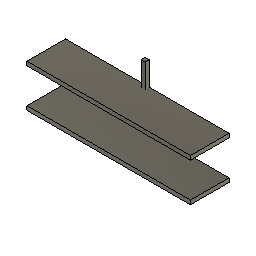
model (Autodesk Fusion 360 design; units mm, degrees)
Autodesk Fusion 360 part; units mm, degrees
sketch "front" plane through (0, 0, 0) normal (0, 1, 0) x (1, 0, 0) in component "shelf"
  line L0 (-10.5, -323.6094) -> (10.5, -323.6094)
  line L1 (10.5, -323.6094) -> (10.5, 200)
  line L2 (10.5, 200) -> (-10.5, 200)
  line L3 (-10.5, 200) -> (-10.5, -323.6094)
  line L4 (-423.6, -200) -> (423.6, -200)
  line L5 (423.6, -200) -> (423.6, -179)
  line L6 (423.6, -179) -> (-423.6, -179)
  line L7 (-423.6, -179) -> (-423.6, -200)
  line L8 (-423.6, 0) -> (423.6, 0)
  line L9 (423.6, 0) -> (423.6, 21)
  line L10 (423.6, 21) -> (-423.6, 21)
  line L11 (-423.6, 21) -> (-423.6, 0)
  line L12 (0, -200) -> (0, 0) construction
  line L13 (0, 0) -> (0, 200) construction
  line L14 (0, -200) -> (0, -323.6094) construction
  arc A0 (-180.0959, 31.5) -> (-217.05, 21) centre (-171.2117, -70.0461) ccw
  arc A1 (-99.149, 38.5819) -> (-10.5, 110.5) centre (-108.0332, 140.128) ccw
  line L15 (-180.0959, 31.5) -> (-99.149, 38.5819)
  line L16 (-10.5, 110.5) -> (10.5, 21) construction
  line L17 (-10.5, 110.5) -> (10.5, 200) construction
  line L18 (-423.6, 0) -> (-217.05, 21) construction
  line L19 (-10.5, 0) -> (-217.05, 21) construction
  arc A2 (-180.0959, -168.5) -> (-217.05, -179) centre (-171.2117, -270.0461) ccw
  line L20 (-180.0959, -168.5) -> (-99.149, -161.4181)
  arc A3 (-99.149, -161.4181) -> (-10.5, -89.5) centre (-108.0332, -59.872) ccw
  arc A4 (217.05, -179) -> (180.0959, -168.5) centre (171.2117, -270.0461) ccw
  line L21 (180.0959, -168.5) -> (99.149, -161.4181)
  arc A5 (10.5, -89.5) -> (99.149, -161.4181) centre (108.0332, -59.872) ccw
  arc A6 (217.05, 21) -> (180.0959, 31.5) centre (171.2117, -70.0461) ccw
  arc A7 (10.5, 110.5) -> (99.149, 38.5819) centre (108.0332, 140.128) ccw
  line L22 (180.0959, 31.5) -> (99.149, 38.5819)
  dimension "d1" = 200
  dimension "d2" = 123.6094
  dimension "d5" = 847.2
  dimension "d7" = 523.6094
  dimension "d9" = 21
  dimension "d11" = 101.934
  dimension "d12" = 5
  dimension "d13" = 10.5
  dimension "d16" = 0
  dimension "d19" = 21
  constraint horizontal L0
  constraint vertical L1
  constraint horizontal L2
  constraint vertical L3
  constraint horizontal L4
  constraint vertical L5
  constraint horizontal L6
  constraint vertical L7
  constraint horizontal L8
  constraint vertical L9
  constraint horizontal L10
  constraint vertical L11
  constraint midpoint L4 L12.start
  constraint midpoint L8 L12.end
  constraint midpoint L2 L13.end
  constraint vertical L12
  constraint vertical L13
  constraint equal L7 L11
  constraint midpoint L0 L14.end
  constraint equal L4 L8
  constraint equal L12 L13
  constraint coincident L12.end L13.start
  constraint coincident L10 A0.end
  constraint coincident L3 A1.end
  constraint tangent A0 L15
  constraint tangent A1 L15
  constraint equal A0 A1
  constraint coincident L1 L16.end
  constraint coincident L10 L16.end
  constraint equal L16 L17
  constraint coincident L3 L19.start
  constraint coincident L8 L19.start
  constraint equal L18 L19
  constraint symmetric L12 A0.end A6.start
  constraint symmetric L12 A0.start A6.end
  constraint symmetric L12 A0 A6
  constraint symmetric L12 A1.end A7.start
  constraint symmetric L12 A1.start A7.end
  constraint symmetric L12 A1 A7
  constraint symmetric L12 A2.start A4.end
  constraint symmetric L12 A2.end A4.start
  constraint symmetric L12 A2 A4
  constraint symmetric L12 L20.end L21.end
  constraint symmetric L12 A3.end A5.start
  constraint symmetric L12 A3 A5
  measures "d1" distance of L12.start L12.end
  measures "d2" distance of L12.start L14.end
  measures "d5" distance of L8.start L8.end
  measures "d7" distance of L0.end L1.end
  measures "d9" distance of L0.start L0.end
  measures "d11" radius of A0
  measures "d12" angle of L10 L15
  measures "d13" distance of L10 A0.start
  measures "d19" distance of L4.start L6.end
extrude "Extrude1" add sketch "front" against normal blind 21 contours L3 L6 A2 L20 A3 | L1 L6 A4 L21 A5 | L3 L10 A0 A1 L15 | L1 L10 A6 A7 L22 makes body 1 at (29.0386, 0, 148.8952) makes body 2 at (-29.0386, 0, -51.1048) makes body 3 at (-29.0386, 0, 148.8952) makes body 4 at (29.0386, 0, -51.1048) in component "shelf"
extrude "Extrude2" add sketch "front" against normal blind 200 separate body contours L3 L4 L6 L7 | L1 L3 L4 L6 | L1 L4 L5 L6 | L3 L8 L10 L11 | L1 L3 L8 L10 | L1 L8 L9 L10 makes body 5 at (141.2, -66.6667, 179) makes body 6 at (141.2, -133.3333, -21) in component "shelf"
extrude "Extrude3" add sketch "front" against normal up to surface (21 mm away) separate body contours L0 L1 L3 L4 | L1 L3 L4 L6 | L1 L3 L6 L8 | L1 L3 L8 L10 | L1 L2 L3 L10 makes body 7 in component "shelf"
sketch "side" plane through (-10.5, 0, 0) normal (-1, 0, 0) x (0, -1, 0) in component "shelf"
  line L0 (21, -200) -> (21, 323.6094)
  line L1 (21, 323.6094) -> (0, 323.6094)
  line L2 (0, 323.6094) -> (0, -200)
  line L3 (0, -200) -> (21, -200)
  arc A0 (110.8669, 165.7722) -> (21, 89.5) centre (119.751, 64.2261) ccw
  line L4 (110.8669, 165.7722) -> (142.0459, 168.5)
  line L5 (0, 179) -> (200, 179)
  line L6 (0, 179) -> (21, 89.5) construction
  line L7 (0, 0) -> (21, 89.5) construction
  arc A1 (142.0459, 168.5) -> (179, 179) centre (133.1617, 270.0461) ccw
  line L8 (0, 179) -> (0, 200)
  line L9 (21, 179) -> (179, 179)
  line L10 (21, -21) -> (179, -21)
  arc A2 (142.0459, -31.5) -> (179, -21) centre (133.1617, 70.0461) ccw
  line L11 (110.8669, -34.2278) -> (142.0459, -31.5)
  arc A3 (110.8669, -34.2278) -> (21, -110.5) centre (119.751, -135.7739) ccw
  point P0 (200, 179)
  dimension "d26" = 101.934
  dimension "d27" = 10.5
  dimension "d29" = 5
  dimension "d31" = 179
  dimension "d34" = 0
  constraint coincident L0 A0.end
  constraint tangent A0 L4
  constraint coincident L5.start L6.start
  constraint coincident L7.start origin
  constraint equal L6 L7
  constraint coincident L5 A1.end
  constraint tangent L4 A1
  constraint equal A0 A1
  constraint coincident L5 L9.start
  constraint coincident L0 L9.start
  measures "d26" radius of A0
  measures "d27" vertical distance of L4.end P0
  measures "d29" angle of L4 L5
  measures "d31" distance of A1.end L8
extrude "Extrude4" add sketch "side" against normal blind 21 separate body contours L0 L10 A2 L11 A3 | L0 A0 L4 L5 A1 L9 makes body 8 at (-10.5, -42.964, 154.1735) makes body 9 at (-10.5, -42.964, -45.8265) in component "shelf"
component "shelf" placed x (1, 0, 0) y (0, 1, 0) z (0, 0, 1) at (0, 0, 0)
equation "d1 = shelfUnit"
equation "d2 = shelfUnit / ratio"
equation "shelfUnit = 200 mm"
equation "d5 = d7 * ratio"
equation "ratio = 1.618"
equation "fourQ = 21 mm"
equation "d9 = fourQ"
equation "supportRadius = fourQ * 3 * ratio"
equation "d11 = supportRadius"
equation "d13 = fourQ / 2"
equation "d17 = -shelfUnit"
equation "d19 = fourQ"
equation "d20 = -fourQ"
equation "d22 = -shelfDepth"
equation "d26 = supportRadius"
equation "d27 = fourQ / 2"
equation "shelfDepth = 200 mm"
equation "d31 = shelfDepth - fourQ"
equation "d35 = -shelfUnit"
equation "d36 = -fourQ"
